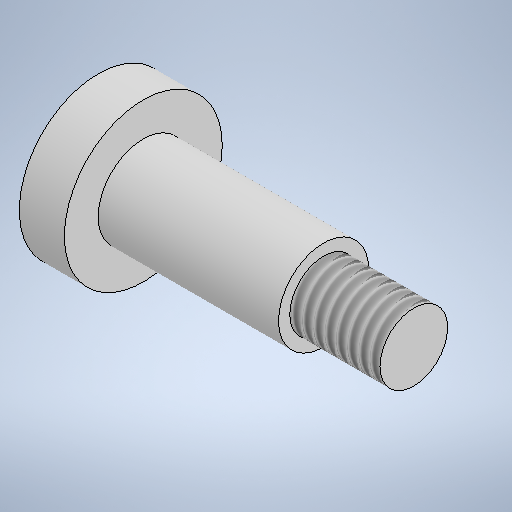
# Autodesk Inventor part: 1 part ß3
Saved by Autodesk Inventor 2025 (Build 290162010, 162A)
## iProperties
Created: 2024-07-30
Part Number: 1 part ß3
Material: Generic
Document SubType Name: Modeling
Designer: Fabri
Density: 1 g/cm^3
Appearance: Default
Author: Fabri
Autodesk Inventor part; units mm, degrees
ref_plane "YZ Plane" through (0, 0, 0) normal (1, 0, 0) x (0, 1, 0)
ref_plane "XZ Plane" through (0, 0, 0) normal (0, 1, 0) x (-1, 0, 0)
ref_plane "XY Plane" through (0, 0, 0) normal (0, 0, 1) x (1, 0, 0)
sketch "Sketch1" plane through (0, 0, 0) normal (0, 0, 1) x (1, 0, 0)
  line L0 (0, 0) -> (0, 3.5)
  line L1 (0, 3.5) -> (2, 3.5)
  line L2 (2, 3.5) -> (2, 2)
  line L3 (2, 2) -> (10, 2)
  line L4 (10, 2) -> (10, 1.5)
  line L5 (10, 1.5) -> (14, 1.5)
  line L6 (14, 1.5) -> (14, 0)
  line L7 (14, 0) -> (0, 0)
  dimension "d0" = 2
  dimension "d1" = 8
  dimension "d2" = 4
  dimension "d3" = 3
  dimension "d4" = 4
  dimension "d5" = 7
  constraints: 16 end point, 7 perpendicular, 1 vertical
  measures "d0" distance of L0.end L1.end
  measures "d1" distance of L2.end L3.end
  measures "d2" distance of L4.end L5.end
  measures "d3" diameter of L5 L7
  measures "d4" diameter of L3 L7
  measures "d5" diameter of L1 L7
revolve "Revolution1" add sketch "Sketch1" angle 360 about axis through (14, 0, 0) along (-1, 0, 0)
thread "Thread1" size "M3x0.5" class "6g" standard "ISO Metric profile" full length
body "Solid1"
